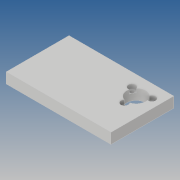
# Autodesk Inventor part: attache_moteur
Saved by Autodesk Inventor 2019 (Build 230136000, 136)
## iProperties
Created: 2020-07-07
Part Number: attache_moteur
Material: Générique
Document SubType Name: Modeling
Designer: Theo
Density: 1 g/cm^3
Appearance: Par défaut
Author: Theo
Autodesk Inventor part; units mm, degrees
ref_plane "YZ Plane" through (0, 0, 0) normal (1, 0, 0) x (0, 1, 0)
ref_plane "XZ Plane" through (0, 0, 0) normal (0, 1, 0) x (-1, 0, 0)
ref_plane "XY Plane" through (0, 0, 0) normal (0, 0, 1) x (1, 0, 0)
sketch "Esquisse1" plane through (0, 0, 0) normal (0, 1, 0) x (-1, 0, 0)
  line L0 (0, 0) -> (100, 0)
  line L1 (100, 0) -> (100, 60)
  line L2 (100, 60) -> (0, 60)
  line L3 (0, 60) -> (0, 0)
  dimension "d1" = 100
  dimension "d2" = 60
  constraints: 8 end point, 2 parallel, 1 horizontal, 1 perpendicular
  measures "d1" distance of L0.start L0.end
  measures "d2" distance of L2.end L0.start
extrude "Extrusion1" add sketch "Esquisse1" along normal blind 10
sketch "Esquisse2" plane through (0, 10, 0) normal (0, 1, 0) x (1, 0, 0)
  circle A0 centre (-18, -18) radius 9
  line L0 (0, 0) -> (-100, 0) projected
  line L1 (-100, 0) -> (-100, -60) projected
  line L2 (-100, -60) -> (0, -60) projected
  line L3 (0, -60) -> (0, 0) projected
  line L4 (-29, -9) -> (-7, -9) construction
  line L5 (-7, -9) -> (-7, -56) construction
  line L6 (-7, -56) -> (-29, -56) construction
  line L7 (-29, -56) -> (-29, -9) construction
  dimension "d5" = 18
  dimension "d7" = 18
  dimension "d9" = 18
  dimension "d27" = 22
  dimension "d28" = 11
  dimension "d29" = 9
  dimension "d30" = 47
  dimension "d31" = 7
  constraints: 8 end point, 2 parallel, 1 centre point, 1 horizontal, 1 perpendicular
  measures "d5" diameter of A0
  measures "d7" distance from line of L3 A0.centre
  measures "d9" distance from line of A0.centre L0
  measures "d27" distance of L4.start L4.end
  measures "d28" horizontal distance of L4.end A0.centre
  measures "d29" distance from line of L4 A0.centre
  measures "d30" distance of L6.end L4.start
  measures "d31" distance between parallel lines of L3 L5
extrude "Extrusion2" cut sketch "Esquisse2" against normal up to surface (10 mm away) contours A0
sketch "Esquisse4" plane through (0, 10, 0) normal (0, 1, 0) x (1, 0, 0)
  circle A0 centre (-18, -18) radius 9 projected
  line L0 (0, 0) -> (-100, 0) projected
  line L1 (-100, 0) -> (-100, -60) projected
  line L2 (-100, -60) -> (0, -60) projected
  line L3 (0, -60) -> (0, 0) projected
  point P0 (-18, -29)
  dimension "d16" = 11
  constraints: 1 vertical alignment
  measures "d16" distance of point (-18, -29) A0.centre
hole "Perçage1" at (-18, 10, 29) direction (0, -1, 0) diameter 3.4 end through all counterbore diameter 7 counterbore depth 4 clearance for "Vis d'assemblage à tête hexagonale ISO 24017" size "M3" standard "ISO"
pattern_circular "Réseau circulaire1" count 3 over 360 about axis through (-18, 10, 18) along (0, -1, 0) of "Perçage1"
equation "\"d28\" = 0.5 * d27"
